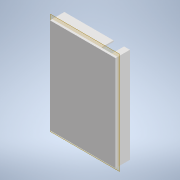
# Autodesk Inventor part: Buttom Plate
Saved by Autodesk Inventor 2020 (Build 240168000, 168)
## iProperties
Created: 2019-11-08
Part Number: Buttom Plate
Material: Generic
Document SubType Name: Modeling
Designer: siwat
Density: 1 g/cm^3
Appearance: Default
Author: siwat
Autodesk Inventor part; units mm, degrees
ref_plane "YZ Plane" through (0, 0, 0) normal (1, 0, 0) x (0, 1, 0)
ref_plane "XZ Plane" through (0, 0, 0) normal (0, 1, 0) x (-1, 0, 0)
ref_plane "XY Plane" through (0, 0, 0) normal (0, 0, 1) x (1, 0, 0)
ref_plane "Work Plane1" through (0, 0, 0) normal (0, 0, 1) x (1, 0, 0)
sketch "Sketch1" plane through (0, 0, 0) normal (0, 0, 1) x (1, 0, 0)
  line L0 (38.904, 56.6039) -> (-39.0955, 56.6039)
  line L1 (-39.0955, 56.6039) -> (-39.0955, -56.8569)
  line L2 (-39.0955, -56.8569) -> (38.904, -56.8569)
  line L3 (38.904, -56.8569) -> (38.904, 56.6039)
  line L4 (-37.4141, -55.0738) -> (37.4715, -55.0738)
  line L5 (37.4715, -55.0738) -> (37.4715, 55.1115)
  line L6 (37.4715, 55.1115) -> (-37.4141, 55.1115)
  line L7 (-37.4141, 55.1115) -> (-37.4141, -55.0738)
  point P0 (0, 0)
  constraints: 16 end point, 4 parallel, 2 horizontal, 2 perpendicular
extrude "Extrusion1" add sketch "Sketch1" along normal blind 2.0625 and the other way blind 14.525
sketch "Sketch2" plane through (0, 0, 2.0625) normal (0, 0, 1) x (1, 0, 0)
  line L0 (38.904, 56.6039) -> (-39.0955, 56.6039)
  line L1 (-39.0955, 56.6039) -> (-39.0955, -56.8569)
  line L2 (-39.0955, -56.8569) -> (38.904, -56.8569)
  line L3 (38.904, -56.8569) -> (38.904, 56.6039)
  point P0 (0, 0)
  constraints: 8 end point, 2 parallel, 1 horizontal, 1 perpendicular
extrude "Extrusion2" add sketch "Sketch2" along normal blind 0.59
sketch "Sketch3" plane through (-39.0955, -56.8569, -14.525) normal (-1, 0, 0) x (0, 0, 1)
  line L0 (14.525, 65.2907) -> (0, 65.2907)
  line L1 (0, 65.2907) -> (0, 84.283)
  line L2 (0, 84.283) -> (14.525, 84.283)
  line L3 (14.525, 84.283) -> (14.525, 65.2907)
  line L4 (0, 0) -> (0, 113.4608) projected
  point P0 (14.525, 56.8569)
  constraints: 8 end point, 2 parallel, 1 horizontal, 1 perpendicular, 1 point on line
extrude "Extrusion3" cut sketch "Sketch3" against normal up to surface (1.6814 mm away)
sketch "Sketch4" plane through (-39.0955, 56.6039, -14.525) normal (0, 1, 0) x (1, 0, 0)
  line L0 (77.9995, 0) -> (0, 0) projected
  line L1 (58.5885, -14.525) -> (71.0413, -14.525)
  line L2 (71.0413, -14.525) -> (71.0413, 0)
  line L3 (71.0413, 0) -> (58.5885, 0)
  line L4 (58.5885, 0) -> (58.5885, -14.525)
  point P0 (39.0955, -14.525)
  constraints: 8 end point, 2 parallel, 1 horizontal, 1 perpendicular, 1 point on line
extrude "Extrusion4" cut sketch "Sketch4" against normal up to surface (1.4924 mm away)
sketch "Sketch6" plane through (0, 0, 2.0625) normal (0, 0, -1) x (-1, 0, 0)
  line L0 (35.9141, -53.5738) -> (-35.9715, -53.5738)
  line L1 (-35.9715, -53.5738) -> (-35.9715, 53.6115)
  line L2 (-35.9715, 53.6115) -> (35.9141, 53.6115)
  line L3 (35.9141, 53.6115) -> (35.9141, -53.5738)
  line L4 (-37.4715, 55.1115) -> (-31.9458, 55.1115) projected
  line L5 (-37.4715, -55.0738) -> (-37.4715, 55.1115) projected
  line L6 (37.4141, -55.0738) -> (-37.4715, -55.0738) projected
  line L7 (37.4141, 8.4338) -> (37.4141, -55.0738) projected
  line L8 (37.4141, -55.0738) -> (37.4141, 55.1115) projected
  line L9 (-37.4715, 55.1115) -> (-37.4715, -55.0738) projected
  line L10 (37.4141, -55.0738) -> (-37.4715, -55.0738)
  line L11 (-37.4715, -55.0738) -> (-37.4715, 55.1115)
  line L12 (-37.4715, 55.1115) -> (37.4141, 55.1115)
  line L13 (37.4141, 55.1115) -> (37.4141, -55.0738)
  point P0 (0, 0)
  dimension "d12" = 1.5
  dimension "d13" = 1.5
  dimension "d14" = 1.5
  dimension "d15" = 1.5
  constraints: 16 end point, 4 parallel, 2 horizontal, 2 perpendicular
  measures "d12" distance between parallel lines of L2 L4
  measures "d13" distance between parallel lines of L5 L1
  measures "d14" distance between parallel lines of L6 L0
  measures "d15" distance between parallel lines of L7 L3
extrude "Extrusion6" add sketch "Sketch6" along normal up to surface (2.0625 mm away)
sketch "Sketch5" plane through (0, 0, 2.0625) normal (0, 0, -1) x (-1, 0, 0)
  circle A0 centre (33.0429, -48.5316) radius 1.6001
  circle A1 centre (11.8743, 21.7468) radius 1.6087
  circle A2 centre (-29.2374, 31.3404) radius 1.6463
  circle A3 centre (-15.7576, -8.1834) radius 1.5639
  circle A4 centre (-29.803, -47.9298) radius 1.5995
  point P0 (0, 0)
  constraints: 5 centre point
extrude "Extrusion5" add sketch "Sketch5" along normal blind 4.5
body "Solid1"
